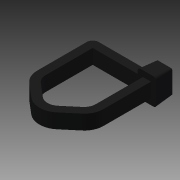
# Autodesk Inventor part: fastener_02
Saved by Autodesk Inventor 2013 (Build 170138000, 138)
## iProperties
Created: 2014-03-16
Part Number: fastener_02
Document SubType Name: Modeling
Designer: Noa Izumi
Material: Default
Density: 1 g/cm^3
Control State: 0
Master: False
Checked Out: False
Shininess: 41.0
Density: 0.0
Volumn: 0.0
Area: 0.0
PropertySet Name: Model Information
Author: Noa Izumi
Autodesk Inventor part; units mm, degrees
ref_plane "YZ Plane" through (0, 0, 0) normal (1, 0, 0) x (0, 1, 0)
ref_plane "XZ Plane" through (0, 0, 0) normal (0, 1, 0) x (-1, 0, 0)
ref_plane "XY Plane" through (0, 0, 0) normal (0, 0, 1) x (1, 0, 0)
sketch "Sketch1" plane through (0, 0, 0) normal (0, 0, 1) x (1, 0, 0)
  line L0 (-0.1, 3.0255) -> (8.5, 3.0255)
  line L1 (8.5, 3.0255) -> (8.5, -5.0485)
  line L2 (-0.1, -5.0485) -> (-0.1, 3.0255)
  arc A0 (2.9061, -8.525) -> (5.4939, -8.525) centre (4.2, -7) ccw
  line L3 (0.6061, -6.5735) -> (2.9061, -8.525)
  line L4 (7.7939, -6.5735) -> (5.4939, -8.525)
  arc A1 (-0.1, -5.0485) -> (0.6061, -6.5735) centre (1.9, -5.0485) ccw
  arc A2 (8.7584, -7.5913) -> (9.8881, -5.1512) centre (6.6881, -5.1512) ccw
  line L5 (8.7584, -7.5913) -> (6.3997, -9.5925)
  arc A3 (2.0003, -9.5925) -> (6.3997, -9.5925) centre (4.2, -7) ccw
  line L6 (2.0003, -9.5925) -> (-0.2997, -7.6411)
  arc A4 (-1.5, -5.0485) -> (-0.2997, -7.6411) centre (1.9, -5.0485) ccw
  line L7 (-1.5, -5.0485) -> (-1.5, 3.4255)
  line L8 (-0.5, 4.4255) -> (9.8881, 4.4255)
  line L9 (9.8881, 4.4255) -> (9.8881, -5.1512)
  arc A5 (-0.5, 4.4255) -> (-1.5, 3.4255) centre (-0.5, 3.4255) ccw
  arc A6 (7.7939, -6.5735) -> (8.5, -5.0485) centre (6.5, -5.0485) ccw
  point P0 (-0.1, -5.9745)
  dimension "d1" = 9
  dimension "d2" = 4
  dimension "d4" = 2
  dimension "d5" = 1.4
  dimension "d6" = 1
  dimension "d16" = 2
  dimension "d19" = 8.6
  dimension "d20" = 2.3
  constraints: 20 end point, 14 point on circle, 14 tangent, 7 centre point, 2 parallel, 2 perpendicular, 2 point on line, 1 horizontal, 4 other
  measures "d1" distance of point (-0.1, -5.974) L0.start
  measures "d2" diameter of A0
  measures "d4" radius of A1
  measures "d5" distance between parallel lines of L5 L4
  measures "d6" radius of A5
  measures "d16" radius of A6
  measures "d19" distance between parallel lines of L1 L2
  measures "d20" horizontal distance of A0.centre A1.centre
extrude "Extrusion1" add sketch "Sketch1" along normal blind 2.5
sketch "Sketch2" plane through (-0.1, 3.0255, 2.5) normal (0, -1, 0) x (1, 0, 0)
  line L0 (8.2, 1) -> (10.4, 1)
  line L1 (10.9, 0.5) -> (10.9, -3)
  line L2 (10.4, -3.5) -> (8.2, -3.5)
  line L3 (7.7, -3) -> (7.7, 0.5)
  arc A0 (8.2, 1) -> (7.7, 0.5) centre (8.2, 0.5) ccw
  arc A1 (10.9, 0.5) -> (10.4, 1) centre (10.4, 0.5) ccw
  arc A2 (10.4, -3.5) -> (10.9, -3) centre (10.4, -3) ccw
  arc A3 (7.7, -3) -> (8.2, -3.5) centre (8.2, -3) ccw
  line L4 (-1.4, -2.5) -> (-1.4, 0) projected
  point P0 (7.7, 1)
  point P1 (10.9, -3.5)
  point P2 (10.9, 1)
  dimension "d9" = 4.5
  dimension "d10" = 3.2
  dimension "d13" = 0.5
  dimension "d21" = 9.1
  constraints: 8 end point, 8 point on circle, 8 tangent, 6 point on line, 4 centre point, 3 equal radius, 2 parallel, 1 horizontal, 1 perpendicular
  measures "d9" distance of point (10.9, 1) point (10.9, -3.5)
  measures "d10" distance of point (7.7, 1) point (10.9, 1)
  measures "d13" radius of A0
  measures "d21" distance between parallel lines of L3 L4
extrude "Extrusion2" add sketch "Sketch2" against normal blind 3 draft -5
